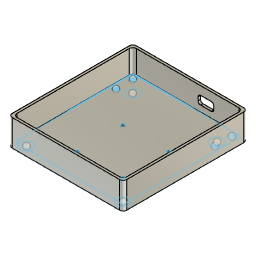
Plaid-Pad Case MX Hi-Pro Simple (Autodesk Fusion 360 design; units mm, degrees)
Autodesk Fusion 360 part; units mm, degrees
sketch "pcb" plane through (0, 0, 0) normal (0, 0, 1) x (1, 0, 0)
  line L0 (90.0735, 95.5726) -> (90.0735, 2.573)
  spline S0 degree 3 poles (90.075, 95.5706) (90.075, 96.9513) (88.9557, 98.0706) (87.575, 98.0706) (87.575, 98.0706) (87.5749, 98.0706) (87.5749, 98.0706) knots 0 0 0 0 1 1 1 2 2 2 2
  spline S1 degree 3 poles (87.5749, 0.0706) (88.9556, 0.0706) (90.0749, 1.1898) (90.075, 2.5705) knots 0 0 0 0 1 1 1 1
  spline S2 degree 3 poles (4.075, 95.1706) (4.6825, 95.1706) (5.175, 94.6781) (5.175, 94.0706) (5.175, 93.4631) (4.6825, 92.9706) (4.075, 92.9706) (3.4675, 92.9706) (2.975, 93.4631) (2.975, 94.0706) (2.975, 94.6781) (3.4675, 95.1706) (4.075, 95.1706) knots 0 0 0 0 1 1 1 2 2 2 3 3 3 4 4 4 4
  line L1 (87.5741, 98.0719) -> (2.573, 98.0719)
  spline S3 degree 3 poles (4.075, 81.1706) (4.6825, 81.1706) (5.175, 80.6781) (5.175, 80.0706) (5.175, 79.4631) (4.6825, 78.9706) (4.075, 78.9706) (3.4675, 78.9706) (2.975, 79.4631) (2.975, 80.0706) (2.975, 80.6781) (3.4675, 81.1706) (4.075, 81.1706) knots 0 0 0 0 1 1 1 2 2 2 3 3 3 4 4 4 4
  spline S4 degree 3 poles (86.075, 81.1706) (86.6825, 81.1706) (87.175, 80.6781) (87.175, 80.0706) (87.175, 79.4631) (86.6825, 78.9706) (86.075, 78.9706) (85.4675, 78.9706) (84.975, 79.4631) (84.975, 80.0706) (84.975, 80.6781) (85.4675, 81.1706) (86.075, 81.1706) knots 0 0 0 0 1 1 1 2 2 2 3 3 3 4 4 4 4
  spline S5 degree 3 poles (71.075, 20.1706) (71.6826, 20.1706) (72.175, 19.6781) (72.175, 19.0706) (72.175, 18.4631) (71.6826, 17.9706) (71.075, 17.9706) (70.4675, 17.9706) (69.975, 18.4631) (69.975, 19.0706) (69.975, 19.6781) (70.4675, 20.1706) (71.075, 20.1706) knots 0 0 0 0 1 1 1 2 2 2 3 3 3 4 4 4 4
  line L2 (87.5741, 0.0711) -> (2.573, 0.0711)
  spline S6 degree 3 poles (33.0751, 58.1705) (33.6826, 58.1705) (34.1751, 57.678) (34.1751, 57.0705) (34.1751, 56.463) (33.6826, 55.9705) (33.0751, 55.9705) (32.4676, 55.9705) (31.9751, 56.463) (31.9751, 57.0705) (31.9751, 57.678) (32.4676, 58.1705) (33.0751, 58.1705) knots 0 0 0 0 1 1 1 2 2 2 3 3 3 4 4 4 4
  spline S7 degree 3 poles (86.075, 95.1706) (86.6825, 95.1706) (87.175, 94.6781) (87.175, 94.0706) (87.175, 93.4631) (86.6825, 92.9706) (86.075, 92.9706) (85.4675, 92.9706) (84.975, 93.4631) (84.975, 94.0706) (84.975, 94.6781) (85.4675, 95.1706) (86.075, 95.1706) knots 0 0 0 0 1 1 1 2 2 2 3 3 3 4 4 4 4
  spline S8 degree 3 poles (0.075, 2.5705) (0.0751, 1.1898) (1.1943, 0.0706) (2.575, 0.0706) knots 0 0 0 0 1 1 1 1
  line L3 (0.0737, 2.573) -> (0.0737, 95.5726)
  spline S9 degree 3 poles (71.075, 58.1705) (71.6826, 58.1705) (72.175, 57.678) (72.175, 57.0705) (72.175, 56.463) (71.6826, 55.9705) (71.075, 55.9705) (70.4675, 55.9705) (69.975, 56.463) (69.975, 57.0705) (69.975, 57.678) (70.4675, 58.1705) (71.075, 58.1705) knots 0 0 0 0 1 1 1 2 2 2 3 3 3 4 4 4 4
  spline S10 degree 3 poles (2.575, 98.0706) (1.1943, 98.0706) (0.075, 96.9513) (0.075, 95.5706) knots 0 0 0 0 1 1 1 1
  spline S11 degree 3 poles (33.0751, 20.1706) (33.6826, 20.1706) (34.1751, 19.6781) (34.1751, 19.0706) (34.1751, 18.4631) (33.6826, 17.9706) (33.0751, 17.9706) (32.4676, 17.9706) (31.9751, 18.4631) (31.9751, 19.0706) (31.9751, 19.6781) (32.4676, 20.1706) (33.0751, 20.1706) knots 0 0 0 0 1 1 1 2 2 2 3 3 3 4 4 4 4
sketch "Sketch5" plane through (0, 0, 0) normal (0, 0, 1) x (1, 0, 0)
  line L0 (2, 0) -> (88, 0)
  line L1 (90, 2) -> (90, 96)
  line L2 (88, 98) -> (2, 98)
  line L3 (0, 96) -> (0, 2)
  arc A0 (90, 96) -> (88, 98) centre (88, 96) ccw
  arc A1 (2, 98) -> (0, 96) centre (2, 96) ccw
  arc A2 (88, 0) -> (90, 2) centre (88, 2) ccw
  arc A3 (0, 2) -> (2, 0) centre (2, 2) ccw
  line L4 (-0.5, 96) -> (-0.5, 2)
  arc A4 (-0.5, 2) -> (2, -0.5) centre (2, 2) ccw
  line L5 (2, -0.5) -> (88, -0.5)
  arc A5 (88, -0.5) -> (90.5, 2) centre (88, 2) ccw
  line L6 (90.5, 2) -> (90.5, 96)
  arc A6 (90.5, 96) -> (88, 98.5) centre (88, 96) ccw
  line L7 (88, 98.5) -> (2, 98.5)
  arc A7 (2, 98.5) -> (-0.5, 96) centre (2, 96) ccw
  point P0 (90, 0)
  point P1 (90, 98)
  point P2 (0, 98)
  dimension "d63" = 98
  dimension "d64" = 90
  dimension "d65" = 2
  dimension "d66" = 2
  dimension "d67" = 2
  dimension "d68" = 2
  dimension "d69" = 0.5
  constraint horizontal L0
  constraint vertical L1
  constraint horizontal L2
  constraint vertical L3
  constraint coincident P1 L1
  constraint coincident P1 L2
  constraint tangent L1 A0
  constraint tangent L2 A0
  constraint coincident P2 L2
  constraint coincident P2 L3
  constraint tangent L2 A1
  constraint tangent L3 A1
  constraint coincident P0 L0
  constraint coincident P0 L1
  constraint tangent L0 A2
  constraint tangent L1 A2
  constraint tangent L0 A3
  constraint tangent L3 A3
  measures "d63" distance of P0 P1
  measures "d64" distance of P1 P2
  measures "d65" radius of A0
  measures "d66" radius of A1
  measures "d67" radius of A2
  measures "d68" radius of A3
sketch "case" plane through (0, 0, 0) normal (0, 0, 1) x (1, 0, 0)
  line L0 (87.5741, 98.0719) -> (2.573, 98.0719)
  line L1 (0.0737, 2.573) -> (0.0737, 95.5726)
  line L2 (90.0735, 95.5726) -> (90.0735, 2.573)
  line L3 (87.5741, 0.0711) -> (2.573, 0.0711)
  line L4 (90.5735, 98.5719) -> (-0.4263, 98.5719)
  line L5 (-0.4263, -0.4289) -> (-0.4263, 98.5719)
  line L6 (90.5735, 98.5719) -> (90.5735, -0.4289)
  line L7 (90.5735, -0.4289) -> (-0.4263, -0.4289)
  line L8 (-2.4263, -2.4289) -> (-2.4263, 100.5719)
  line L9 (92.5735, 100.5719) -> (-2.4263, 100.5719)
  line L10 (92.5735, 100.5719) -> (92.5735, -2.4289)
  line L11 (92.5735, -2.4289) -> (-2.4263, -2.4289)
  line L12 (-2.4263, 76.3719) -> (92.5735, 76.3719)
  spline S0 degree 3 poles (33.0751, 58.1705) (33.6826, 58.1705) (34.1751, 57.678) (34.1751, 57.0705) (34.1751, 56.463) (33.6826, 55.9705) (33.0751, 55.9705) (32.4676, 55.9705) (31.9751, 56.463) (31.9751, 57.0705) (31.9751, 57.678) (32.4676, 58.1705) (33.0751, 58.1705) knots 0 0 0 0 1 1 1 2 2 2 3 3 3 4 4 4 4
  spline S1 degree 3 poles (33.0751, 20.1706) (33.6826, 20.1706) (34.1751, 19.6781) (34.1751, 19.0706) (34.1751, 18.4631) (33.6826, 17.9706) (33.0751, 17.9706) (32.4676, 17.9706) (31.9751, 18.4631) (31.9751, 19.0706) (31.9751, 19.6781) (32.4676, 20.1706) (33.0751, 20.1706) knots 0 0 0 0 1 1 1 2 2 2 3 3 3 4 4 4 4
  spline S2 degree 3 poles (71.075, 58.1705) (71.6826, 58.1705) (72.175, 57.678) (72.175, 57.0705) (72.175, 56.463) (71.6826, 55.9705) (71.075, 55.9705) (70.4675, 55.9705) (69.975, 56.463) (69.975, 57.0705) (69.975, 57.678) (70.4675, 58.1705) (71.075, 58.1705) knots 0 0 0 0 1 1 1 2 2 2 3 3 3 4 4 4 4
  spline S3 degree 3 poles (71.075, 20.1706) (71.6826, 20.1706) (72.175, 19.6781) (72.175, 19.0706) (72.175, 18.4631) (71.6826, 17.9706) (71.075, 17.9706) (70.4675, 17.9706) (69.975, 18.4631) (69.975, 19.0706) (69.975, 19.6781) (70.4675, 20.1706) (71.075, 20.1706) knots 0 0 0 0 1 1 1 2 2 2 3 3 3 4 4 4 4
  spline S4 degree 3 poles (4.075, 81.1706) (4.6825, 81.1706) (5.175, 80.6781) (5.175, 80.0706) (5.175, 79.4631) (4.6825, 78.9706) (4.075, 78.9706) (3.4675, 78.9706) (2.975, 79.4631) (2.975, 80.0706) (2.975, 80.6781) (3.4675, 81.1706) (4.075, 81.1706) knots 0 0 0 0 1 1 1 2 2 2 3 3 3 4 4 4 4
  spline S5 degree 3 poles (4.075, 95.1706) (4.6825, 95.1706) (5.175, 94.6781) (5.175, 94.0706) (5.175, 93.4631) (4.6825, 92.9706) (4.075, 92.9706) (3.4675, 92.9706) (2.975, 93.4631) (2.975, 94.0706) (2.975, 94.6781) (3.4675, 95.1706) (4.075, 95.1706) knots 0 0 0 0 1 1 1 2 2 2 3 3 3 4 4 4 4
  spline S6 degree 3 poles (86.075, 95.1706) (86.6825, 95.1706) (87.175, 94.6781) (87.175, 94.0706) (87.175, 93.4631) (86.6825, 92.9706) (86.075, 92.9706) (85.4675, 92.9706) (84.975, 93.4631) (84.975, 94.0706) (84.975, 94.6781) (85.4675, 95.1706) (86.075, 95.1706) knots 0 0 0 0 1 1 1 2 2 2 3 3 3 4 4 4 4
  spline S7 degree 3 poles (86.075, 81.1706) (86.6825, 81.1706) (87.175, 80.6781) (87.175, 80.0706) (87.175, 79.4631) (86.6825, 78.9706) (86.075, 78.9706) (85.4675, 78.9706) (84.975, 79.4631) (84.975, 80.0706) (84.975, 80.6781) (85.4675, 81.1706) (86.075, 81.1706) knots 0 0 0 0 1 1 1 2 2 2 3 3 3 4 4 4 4
  circle A0 centre (71.0751, 57.0704) radius 1.1001
  circle A1 centre (86.0749, 80.0705) radius 1.1001
  circle A2 centre (86.0751, 94.0707) radius 1.1001
  circle A3 centre (4.0751, 80.0706) radius 1.1002
  circle A4 centre (33.0752, 57.0705) radius 1.1002
  circle A5 centre (33.0751, 19.0707) radius 1.1001
  circle A6 centre (71.0751, 19.0704) radius 1.1002
  circle A7 centre (4.0749, 94.0706) radius 2.25
  circle A8 centre (4.0751, 80.0706) radius 2.25
  circle A9 centre (86.0751, 94.0707) radius 2.25
  circle A10 centre (86.0749, 80.0705) radius 2.25
  circle A11 centre (71.0751, 57.0704) radius 2.25
  circle A12 centre (33.0752, 57.0705) radius 2.25
  circle A13 centre (33.0751, 19.0707) radius 2.25
  circle A14 centre (71.0751, 19.0704) radius 2.25
  line L13 (66.0735, 98.5719) -> (66.0735, 94.2441) construction
  line L14 (57.0735, 98.5719) -> (57.0735, 93.9093) construction
  dimension "d5" = 0.5
  dimension "d6" = 0.5
  dimension "d7" = 0.5
  dimension "d8" = 0.5
  dimension "d11" = 2
  dimension "d16" = 21.7
  dimension "d20" = 4.5
  dimension "d21" = 4.5
  dimension "d22" = 4.5
  dimension "d23" = 4.5
  dimension "d24" = 4.5
  dimension "d25" = 4.5
  dimension "d26" = 4.5
  dimension "d27" = 4.5
  dimension "d39" = 33
  dimension "d40" = 24
  constraint parallel L2 L6
  constraint parallel L0 L4
  constraint parallel L1 L5
  constraint parallel L3 L7
  constraint coincident L8 L12.start
  constraint coincident L10 L12.end
  constraint perpendicular L10 L12
  constraint concentric A3 A8
  constraint concentric A2 A9
  constraint concentric A1 A10
  constraint concentric A0 A11
  constraint concentric A4 A12
  constraint concentric A5 A13
  constraint concentric A6 A14
  constraint coincident L4 L13.start
  constraint perpendicular L0 L13
  constraint coincident L4 L14.start
  constraint perpendicular L0 L14
  measures "d5" distance of L0 L4
  measures "d6" distance of L2 L6
  measures "d7" distance of L3 L7
  measures "d8" distance of L1 L5
  measures "d16" distance of L0 L12
  measures "d20" diameter of A7
  measures "d21" diameter of A8
  measures "d22" diameter of A9
  measures "d23" diameter of A10
  measures "d24" diameter of A11
  measures "d25" diameter of A12
  measures "d26" diameter of A13
  measures "d27" diameter of A14
  measures "d39" distance of L2 L14
  measures "d40" distance of L2 L13
extrude "Extrude1" add sketch "case" against normal blind 3 contours L4 L5 L6 L12 | L4 L5 L6 L8 L9 L10 L12 | L5 L6 L7 L8 L10 L11 L12 | L5 L6 L7 L12 | S4 A3 | S5 | S6 A2 | S7 A1 | A7 | A8 | A9 | A10 | A11 | A12 | A13 | A14
extrude "Extrude2" add sketch "case" along normal blind 19 contours L4 L5 L6 L8 L9 L10 L12 | L5 L6 L7 L8 L10 L11 L12
fillet "Fillet5" radius 3 4 edges at (-0.4263, -0.4289, 9.5) (90.5735, -0.4289, 9.5) (90.5735, 98.5719, 9.5) (-0.4263, 98.5719, 9.5)
extrude "Extrude10" cut sketch "case" against normal through all from surface at -1.5 contours A11 | A12 | A13 | A14
sketch "usb" plane through (0, 98.5719, 0) normal (0, -1, 0) x (1, 0, 0)
  line L0 (-0.5263, 0) -> (90.6735, 0)
  line L1 (55.6735, 7) -> (64.6735, 7)
  line L2 (64.6735, 7) -> (64.6735, 10)
  line L3 (64.6735, 10) -> (55.6735, 10)
  line L4 (55.6735, 10) -> (55.6735, 7)
  line L5 (66.6735, 5) -> (66.6735, 12)
  line L6 (66.6735, 12) -> (53.6735, 12)
  line L7 (53.6735, 12) -> (53.6735, 5)
  line L8 (53.6735, 5) -> (66.6735, 5)
  line L9 (90.6735, 0) -> (90.6735, 16.6)
  line L10 (90.6735, 16.6) -> (-0.5263, 16.6)
  line L11 (-0.5263, 16.6) -> (-0.5263, 0)
  line L12 (87.5741, 0) -> (2.573, 0)
  line L13 (88, 17) -> (2, 17)
  line L14 (2, 17) -> (2, 0)
  line L15 (2, 0) -> (88, 0)
  line L16 (88, 0) -> (88, 17)
  line L17 (87.5735, 19) -> (2.5737, 19)
  line L18 (2.5737, 0) -> (87.5735, 0)
  line L19 (2.5737, 19) -> (2.5737, 0)
  line L20 (87.5735, 0) -> (87.5735, 19)
  point P0 (57.0735, 0)
  point P1 (66.0735, 0)
  point P2 (60.1735, 10)
  dimension "d41" = 3
  dimension "d43" = 2
  dimension "d77" = 7
  dimension "d79" = 30.5
  constraint horizontal L1
  constraint vertical L2
  constraint horizontal L3
  constraint vertical L4
  constraint midpoint L3 P2
  measures "d41" distance of L1.start L3.end
  measures "d77" distance of L1 L15
  measures "d79" distance of L9 P2
extrude "Extrude6" cut sketch "usb" against normal through all contours L1 L2 L3 L4 | L5 L6 L7 L8
fillet "Fillet3" radius 2 4 edges at (53.6735, 99.5719, 12) (53.6735, 99.5719, 5) (66.6735, 99.5719, 5) (66.6735, 99.5719, 12)
fillet "Fillet6" radius 3 4 edges at (92.5735, -2.4289, 8) (-2.4263, -2.4289, 8) (92.5735, 100.5719, 8) (-2.4263, 100.5719, 8)
sketch "Sketch6" plane through (0, 0, 0) normal (0, 0, 1) x (1, 0, 0)
  circle A0 centre (4.1, 94.1) radius 2.25
  circle A1 centre (4.1, 80.1) radius 2.25
  circle A2 centre (86.1, 80.1) radius 2.25
  circle A3 centre (86.1, 94.1) radius 2.25
  dimension "d87" = 4.5
  dimension "d88" = 4.5
  dimension "d89" = 4.5
  dimension "d90" = 4.5
  measures "d87" diameter of A0
  measures "d88" diameter of A1
  measures "d89" diameter of A2
  measures "d90" diameter of A3
extrude "Extrude11" cut sketch "Sketch6" against normal blind 1 contours A0
extrude "Extrude12" cut sketch "Sketch6" against normal blind 1 contours A1
extrude "Extrude13" cut sketch "Sketch6" against normal blind 1 contours A3
extrude "Extrude14" cut sketch "Sketch6" against normal blind 1 contours A2
sketch "Sketch7" plane through (0, 0, -3) normal (0, 0, -1) x (1, 0, 0)
  arc A0 (-2.4263, -97.5719) -> (0.5737, -100.5719) centre (0.5737, -97.5719) ccw
  line L0 (0.5737, -100.5719) -> (89.5735, -100.5719)
  arc A1 (89.5735, -100.5719) -> (92.5735, -97.5719) centre (89.5735, -97.5719) ccw
  line L1 (92.5735, -97.5719) -> (92.5735, -0.5711)
  arc A2 (92.5735, -0.5711) -> (89.5735, 2.4289) centre (89.5735, -0.5711) ccw
  line L2 (89.5735, 2.4289) -> (0.5737, 2.4289)
  arc A3 (0.5737, 2.4289) -> (-2.4263, -0.5711) centre (0.5737, -0.5711) ccw
  line L3 (-2.4263, -0.5711) -> (-2.4263, -97.5719)
  circle A4 centre (33.0752, -57.0705) radius 2.25
  circle A5 centre (33.0751, -19.0707) radius 2.25
  circle A6 centre (71.0751, -57.0704) radius 2.25
  circle A7 centre (71.0751, -19.0704) radius 2.25
  circle A8 centre (5, -5) radius 5
  circle A9 centre (85, -5) radius 5
  circle A10 centre (81, -87) radius 5
  circle A11 centre (11, -87) radius 5
  dimension "d99" = 10
  dimension "d100" = 10
  dimension "d101" = 10
  measures "d99" diameter of A8
  measures "d100" diameter of A9
  measures "d101" diameter of A11
extrude "Extrude15" cut sketch "Sketch7" against normal blind 1 contours A8
extrude "Extrude16" cut sketch "Sketch7" against normal blind 1 contours A11
extrude "Extrude17" cut sketch "Sketch7" against normal blind 1 contours A10
extrude "Extrude18" cut sketch "Sketch7" against normal blind 1 contours A9
equation "d5 = innerOffset"
equation "d6 = innerOffset"
equation "d7 = innerOffset"
equation "d8 = innerOffset"
equation "innerOffset = 0.5 mm" comment "Gap between pcb and case"
equation "caseWallThickness = 2 mm" comment "Case side thickness"
equation "d11 = caseWallThickness"
equation "d12 = -bottomThickness"
equation "d14 = innerHeight"
equation "d69 = innerOffset"
equation "d79 = 30 mm + innerOffset"
equation "innerHeight = 19 mm" comment "Ends at bottom of keycaps"
equation "bottomThickness = 3 mm" comment "Case bottom thickness"
